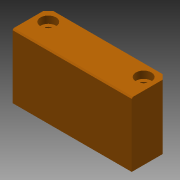
# Autodesk Inventor part: Peripherie_Motor2_liegend
Saved by Autodesk Inventor 2015 (Build 190159000, 159)
## iProperties
Created: 2015-03-02
Part Number: Peripherie_Motor2_liegend
Material: Generisch
Document SubType Name: Modeling
Designer: TowerSebi
Density: 1 g/cm^3
Appearance: Orange
Author: TowerSebi
Autodesk Inventor part; units mm, degrees
ref_plane "YZ Plane" through (0, 0, 0) normal (1, 0, 0) x (0, 1, 0)
ref_plane "XZ Plane" through (0, 0, 0) normal (0, 1, 0) x (-1, 0, 0)
ref_plane "XY Plane" through (0, 0, 0) normal (0, 0, 1) x (1, 0, 0)
sketch "Skizze1" plane through (0, 0, 0) normal (0, 0, 1) x (1, 0, 0)
  line L0 (0, 0) -> (50, 0)
  line L1 (50, 0) -> (50, 15)
  line L2 (50, 15) -> (0, 15)
  line L3 (0, 15) -> (0, 0)
  dimension "d0" = 15
  dimension "d1" = 50
  constraints: 8 end point, 2 parallel, 1 horizontal, 1 perpendicular
  measures "d0" distance of L2.end L0.start
  measures "d1" distance of L0.start L0.end
extrude "Extrusion1" add sketch "Skizze1" along normal blind 27
hole "Bohrung1" at (45, 10, 27) direction (0, 0, -1) diameter 3.4 end through all counterbore diameter 6.5 counterbore depth 3 clearance for "Inbusschraube DIN EN ISO 4762" size "M3" standard "DIN"
hole "Bohrung2" at (5, 10, 27) direction (0, 0, -1) diameter 3.4 end through all counterbore diameter 6.5 counterbore depth 3 clearance for "Inbusschraube DIN EN ISO 4762" size "M3" standard "DIN"
chamfer "Fase1" distance 0.5 angle 45 1 edges at (25, 0, 27)
sketch "Skizze2" plane through (0, 0, 0) normal (0, 0, -1) x (-1, 0, 0)
  line L0 (0, 15) -> (0, 0) projected
  line L1 (-50, 15) -> (0, 15) projected
  line L2 (-50, 0) -> (-50, 15) projected
  line L3 (-40, 15) -> (-10, 15)
  line L4 (-10, 15) -> (-10, 3)
  line L5 (-10, 3) -> (-40, 3)
  line L6 (-40, 3) -> (-40, 15)
  dimension "d25" = 10
  dimension "d26" = 10
  dimension "d27" = 12
  constraints: 8 end point, 2 parallel, 1 horizontal, 1 perpendicular, 1 point on line
  measures "d25" distance between parallel lines of L2 L6
  measures "d26" distance between parallel lines of L0 L4
  measures "d27" distance between parallel lines of L1 L5
extrude "Extrusion2" cut sketch "Skizze2" against normal blind 25.5
chamfer "Fase2" distance 2 angle 45 2 edges at (50, 15, 13.5) (0, 15, 13.5)
